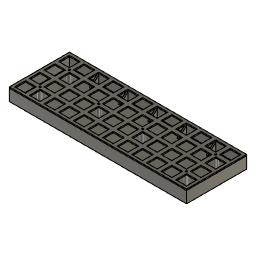
keyboard48 (Autodesk Fusion 360 design; units mm, degrees)
Autodesk Fusion 360 part; units mm, degrees
sketch "Sketch1" plane through (0, 0, 0) normal (0, 0, 1) x (1, 0, 0)
  line L0 (226.5, -3.5) -> (226.5, 74.5)
  line L1 (226.5, 74.5) -> (-3.5, 74.5)
  line L2 (114, 0.05) -> (127.9, 0.05) construction
  line L3 (127.9, 13.95) -> (114, 13.95) construction
  line L4 (223, 64) -> (226.5, 64) construction
  line L5 (206.5, 74.5) -> (206.5, 34.5) construction
  line L6 (199.5, 57.05) -> (213.5, 57.05) construction
  line L7 (213.5, 57.05) -> (213.5, 58.03) construction
  line L8 (213.5, 58.03) -> (215.075, 58.03) construction
  line L9 (215.075, 58.03) -> (215.075, 57.23) construction
  line L10 (215.075, 57.23) -> (216.9, 57.23) construction
  line L11 (216.9, 57.23) -> (216.9, 56.03) construction
  line L12 (216.9, 56.03) -> (219.9, 56.03) construction
  line L13 (219.9, 56.03) -> (219.9, 57.23) construction
  line L14 (219.9, 57.23) -> (221.725, 57.23) construction
  line L15 (221.725, 57.23) -> (221.725, 63.5) construction
  line L16 (221.725, 63.5) -> (222.6, 63.5) construction
  line L17 (222.6, 63.5) -> (222.6, 66.3) construction
  line L18 (222.6, 66.3) -> (221.725, 66.3) construction
  line L19 (221.725, 66.3) -> (221.725, 69.53) construction
  line L20 (221.725, 69.53) -> (215.075, 69.53) construction
  line L21 (215.075, 69.53) -> (215.075, 68.73) construction
  line L22 (215.075, 68.73) -> (213.5, 68.73) construction
  line L23 (213.5, 68.73) -> (213.5, 70.95) construction
  line L24 (213.5, 70.95) -> (199.5, 70.95) construction
  line L25 (199.5, 70.95) -> (199.5, 68.73) construction
  line L26 (199.5, 68.73) -> (197.925, 68.73) construction
  line L27 (197.925, 68.73) -> (197.925, 69.53) construction
  line L28 (197.925, 69.53) -> (191.275, 69.53) construction
  line L29 (191.275, 69.53) -> (191.275, 66.3) construction
  line L30 (190.4, 66.3) -> (190.4, 63.5) construction
  line L31 (190.4, 63.5) -> (191.275, 63.5) construction
  line L32 (191.275, 63.5) -> (191.275, 57.23) construction
  line L33 (191.275, 57.23) -> (193.1, 57.23) construction
  line L34 (193.1, 57.23) -> (193.1, 56.03) construction
  line L35 (193.1, 56.03) -> (196.1, 56.03) construction
  line L36 (196.1, 56.03) -> (196.1, 57.23) construction
  line L37 (196.1, 57.23) -> (197.925, 57.23) construction
  line L38 (197.925, 57.23) -> (197.925, 58.03) construction
  line L39 (197.925, 58.03) -> (199.5, 58.03) construction
  line L40 (199.5, 58.03) -> (199.5, 57.05) construction
  line L41 (190.4, 66.3) -> (191.275, 66.3) construction
  line L42 (199.5, 49.73) -> (197.925, 49.73) construction
  line L43 (215.075, 38.23) -> (216.9, 38.23) construction
  line L44 (213.5, 39.03) -> (215.075, 39.03) construction
  line L45 (213.5, 38.05) -> (213.5, 39.03) construction
  line L46 (215.075, 49.73) -> (213.5, 49.73) construction
  line L47 (213.5, 51.95) -> (199.5, 51.95) construction
  line L48 (199.5, 38.05) -> (213.5, 38.05) construction
  line L49 (193.1, 37.03) -> (196.1, 37.03) construction
  line L50 (191.275, 38.23) -> (193.1, 38.23) construction
  line L51 (197.925, 39.03) -> (199.5, 39.03) construction
  line L52 (222.6, 44.5) -> (222.6, 47.3) construction
  line L53 (221.725, 44.5) -> (222.6, 44.5) construction
  line L54 (199.5, 39.03) -> (199.5, 38.05) construction
  line L55 (191.275, 44.5) -> (191.275, 38.23) construction
  line L56 (196.1, 37.03) -> (196.1, 38.23) construction
  line L57 (221.725, 50.53) -> (215.075, 50.53) construction
  line L58 (196.1, 38.23) -> (197.925, 38.23) construction
  line L59 (215.075, 39.03) -> (215.075, 38.23) construction
  line L60 (197.925, 38.23) -> (197.925, 39.03) construction
  line L61 (197.925, 50.53) -> (191.275, 50.53) construction
  line L62 (216.9, 38.23) -> (216.9, 37.03) construction
  line L63 (191.275, 50.53) -> (191.275, 47.3) construction
  line L64 (190.4, 47.3) -> (191.275, 47.3) construction
  line L65 (199.5, 51.95) -> (199.5, 49.73) construction
  line L66 (197.925, 49.73) -> (197.925, 50.53) construction
  line L67 (219.9, 38.23) -> (221.725, 38.23) construction
  line L68 (215.075, 50.53) -> (215.075, 49.73) construction
  line L69 (193.1, 38.23) -> (193.1, 37.03) construction
  line L70 (219.9, 37.03) -> (219.9, 38.23) construction
  line L71 (221.725, 38.23) -> (221.725, 44.5) construction
  line L72 (190.4, 44.5) -> (191.275, 44.5) construction
  line L73 (190.4, 47.3) -> (190.4, 44.5) construction
  line L74 (222.6, 47.3) -> (221.725, 47.3) construction
  line L75 (213.5, 49.73) -> (213.5, 51.95) construction
  line L76 (216.9, 37.03) -> (219.9, 37.03) construction
  line L77 (221.725, 47.3) -> (221.725, 50.53) construction
  line L78 (114, 13.95) -> (114, 8.45) construction
  line L79 (114, 8.45) -> (94.3177, 8.45) construction
  line L80 (94.3177, 8.45) -> (94.3177, 12.6396) construction
  line L81 (94.3177, 12.6396) -> (87.6629, 12.6396) construction
  line L82 (87.6629, 12.6396) -> (87.6629, 9.244) construction
  line L83 (87.6629, 9.244) -> (86.7993, 9.244) construction
  line L84 (86.7993, 9.244) -> (86.7993, 6.45) construction
  line L85 (86.7993, 6.45) -> (87.6629, 6.45) construction
  line L86 (87.6629, 6.45) -> (87.6629, 0.346) construction
  line L87 (87.6629, 0.346) -> (89.4663, 0.346) construction
  line L88 (89.4663, 0.346) -> (89.4663, -0.8224) construction
  line L89 (89.4663, -0.8224) -> (92.5143, -0.8224) construction
  line L90 (92.5143, -0.8224) -> (92.5143, 0.346) construction
  line L91 (92.5143, 0.346) -> (94.3177, 0.346) construction
  line L92 (94.3177, 0.346) -> (94.3177, 5.45) construction
  line L93 (94.3177, 5.45) -> (114, 5.45) construction
  line L94 (114, 5.45) -> (114, 0.05) construction
  line L95 (127.9, 13.95) -> (127.9, 8.45) construction
  line L96 (127.9, 8.45) -> (147.5823, 8.45) construction
  line L97 (147.5823, 8.45) -> (147.5823, 12.6396) construction
  line L98 (147.5823, 12.6396) -> (154.2371, 12.6396) construction
  line L99 (154.2371, 12.6396) -> (154.2371, 9.244) construction
  line L100 (154.2371, 9.244) -> (155.1007, 9.244) construction
  line L101 (155.1007, 9.244) -> (155.1007, 6.45) construction
  line L102 (155.1007, 6.45) -> (154.2371, 6.45) construction
  line L103 (154.2371, 6.45) -> (154.2371, 0.346) construction
  line L104 (154.2371, 0.346) -> (152.4337, 0.346) construction
  line L105 (152.4337, 0.346) -> (152.4337, -0.8224) construction
  line L106 (152.4337, -0.8224) -> (149.3857, -0.8224) construction
  line L107 (149.3857, -0.8224) -> (149.3857, 0.346) construction
  line L108 (149.3857, 0.346) -> (147.5823, 0.346) construction
  line L109 (147.5823, 0.346) -> (147.5823, 5.45) construction
  line L110 (147.5823, 5.45) -> (127.9, 5.45) construction
  line L111 (127.9, 5.45) -> (127.9, 0.05) construction
  line L112 (71, 6.95) -> (171, 6.95) construction
  line L113 (120.95, 19) -> (120.95, -2.5) construction
  line L114 (90.9903, 16.3311) -> (90.9903, -1.1154) construction
  line L115 (150.9097, 15.5) -> (150.9097, -1.5) construction
  line L116 (86.7993, 9.244) -> (90.9903, 9.244) construction
  line L117 (155.1007, 9.244) -> (150.9097, 9.244) construction
  line L118 (-3.5, 74.5) -> (-3.5, -3.5)
  line L119 (-3.5, -3.5) -> (226.5, -3.5)
  line L120 (0, 0) -> (13.9, 0)
  line L121 (13.9, 0) -> (13.9, 13.9)
  line L122 (13.9, 13.9) -> (0, 13.9)
  line L123 (0, 13.9) -> (0, 0)
  line L124 (-1.5, 72.5) -> (224.5, 72.5)
  line L125 (224.5, 72.5) -> (224.5, -1.5)
  line L126 (224.5, -1.5) -> (-1.5, -1.5)
  line L127 (-1.5, -1.5) -> (-1.5, 72.5)
  dimension "d15" = 14
  dimension "d16" = 6.95
  dimension "d17" = 17.15
  dimension "d18" = 20.8
  dimension "d19" = 26.8
  dimension "d20" = 6.95
  dimension "d21" = 30.45
  dimension "d22" = 32.2
  dimension "d23" = 0.5
  dimension "d24" = 2.3
  dimension "d25" = 5.97
  dimension "d26" = 6.77
  dimension "d27" = 7.97
  dimension "d28" = 4.73
  dimension "d29" = 5.53
  dimension "d32" = 0
  dimension "d33" = -19
  dimension "d34" = 7
  dimension "d35" = 13.9
  dimension "d36" = 13.9
  dimension "d37" = 6.6548
  dimension "d38" = 3.048
  dimension "d39" = 2.794
  dimension "d40" = 4.191
  dimension "d41" = 12.2936
  dimension "d42" = 13.462
  dimension "d43" = 6.604
  dimension "d44" = 0.5
  dimension "d45" = 59.9194
  dimension "d46" = 3
  dimension "d86" = 6.95
  dimension "d87" = 120.95
  dimension "d88" = 20
  dimension "d89" = 10.5
  dimension "d90" = 3.5
  dimension "d91" = 3.5
  dimension "d92" = 230
  dimension "d93" = 78
  dimension "d142" = 13.9
  dimension "d143" = 13.9
  dimension "d155" = 2
  dimension "d156" = 2
  dimension "d157" = 2
  dimension "d158" = 2
  constraint coincident L0 L4.end
  constraint perpendicular L0 L4
  constraint coincident L1 L5.start
  constraint perpendicular L1 L5
  constraint perpendicular L5 L6
  constraint symmetric L5 L6.start L6.end
  constraint perpendicular L6 L7
  constraint perpendicular L7 L8
  constraint perpendicular L8 L9
  constraint perpendicular L9 L10
  constraint perpendicular L10 L11
  constraint perpendicular L11 L12
  constraint perpendicular L10 L13
  constraint perpendicular L13 L14
  constraint perpendicular L14 L15
  constraint perpendicular L13 L16
  constraint perpendicular L4 L17
  constraint perpendicular L17 L18
  constraint perpendicular L4 L19
  constraint perpendicular L19 L20
  constraint vertical L8.end L20.end
  constraint perpendicular L20 L21
  constraint perpendicular L7 L22
  constraint perpendicular L4 L23
  constraint perpendicular L23 L24
  constraint perpendicular L22 L25
  constraint perpendicular L5 L26
  constraint perpendicular L22 L27
  constraint perpendicular L5 L28
  constraint perpendicular L22 L29
  constraint perpendicular L4 L30
  constraint perpendicular L29 L31
  constraint perpendicular L4 L32
  constraint perpendicular L32 L33
  constraint perpendicular L4 L34
  constraint perpendicular L34 L35
  constraint perpendicular L4 L36
  constraint perpendicular L34 L37
  constraint perpendicular L4 L38
  constraint perpendicular L34 L39
  constraint perpendicular L6 L40
  constraint symmetric L5 L9 L38
  constraint symmetric L5 L11 L36
  constraint symmetric L5 L13 L34
  constraint perpendicular L29 L41
  constraint equal L6 L24
  constraint collinear L7 L23
  constraint collinear L27 L38
  constraint collinear L29 L32
  constraint collinear L10 L14
  constraint collinear L8 L39
  constraint collinear L10 L37
  constraint collinear L12 L35
  constraint collinear L14 L33
  constraint collinear L16 L31
  constraint collinear L18 L41
  constraint collinear L20 L28
  constraint collinear L22 L26
  constraint perpendicular L3 L78
  constraint perpendicular L78 L79
  constraint perpendicular L3 L80
  constraint perpendicular L80 L81
  constraint perpendicular L81 L82
  constraint perpendicular L82 L83
  constraint perpendicular L83 L84
  constraint perpendicular L82 L85
  constraint perpendicular L85 L86
  constraint perpendicular L82 L87
  constraint perpendicular L85 L88
  constraint perpendicular L82 L89
  constraint perpendicular L89 L90
  constraint perpendicular L80 L91
  constraint perpendicular L91 L92
  constraint perpendicular L78 L93
  constraint perpendicular L2 L94
  constraint perpendicular L79 L95
  constraint perpendicular L78 L96
  constraint perpendicular L96 L97
  constraint perpendicular L97 L98
  constraint perpendicular L98 L99
  constraint perpendicular L97 L100
  constraint perpendicular L98 L101
  constraint perpendicular L101 L102
  constraint perpendicular L102 L103
  constraint perpendicular L103 L104
  constraint perpendicular L102 L105
  constraint perpendicular L105 L106
  constraint perpendicular L106 L107
  constraint perpendicular L107 L108
  constraint perpendicular L96 L109
  constraint perpendicular L109 L110
  constraint perpendicular L2 L111
  constraint collinear L95 L111
  constraint collinear L78 L94
  constraint collinear L79 L96
  constraint collinear L93 L110
  constraint collinear L82 L86
  constraint collinear L80 L92
  constraint vertical L114
  constraint symmetric L88 L90 L114
  constraint equal L84 L101
  constraint equal L81 L98
  constraint equal L89 L106
  constraint collinear L97 L109
  constraint collinear L99 L103
  constraint coincident L114 L116.end
  constraint perpendicular L114 L116
  constraint coincident L115 L117.end
  constraint perpendicular L115 L117
  constraint equal L116 L117
  constraint collinear L104 L108
  constraint collinear L81 L98
  constraint collinear L91 L108
  constraint collinear L89 L106
  constraint collinear L87 L91
  constraint collinear L85 L102
  constraint symmetric L78 L95 L113
  constraint symmetric L79 L93 L112
  constraint perpendicular L112 L118
  constraint horizontal L1
  constraint symmetric L5 L63 L77
  constraint symmetric L5 L52 L73
  constraint symmetric L5 L55 L71
  constraint horizontal L120
  constraint vertical L121
  constraint horizontal L122
  constraint vertical L123
  constraint coincident L120.start L123.end
  constraint horizontal L124
  constraint vertical L125
  constraint horizontal L126
  constraint vertical L127
  measures "d15" distance of L6.start L6.end
  measures "d16" distance of L4 L6
  measures "d17" distance of L9 L38
  measures "d18" distance of L11 L36
  measures "d19" distance of L13 L34
  measures "d20" distance of L4 L24
  measures "d21" distance of L19 L29
  measures "d22" distance of L17 L30
  measures "d23" distance of L4 L16
  measures "d24" distance of L4 L18
  measures "d25" distance of L4 L8
  measures "d26" distance of L4 L14
  measures "d27" distance of L4 L12
  measures "d28" distance of L4 L22
  measures "d29" distance of L4 L20
  measures "d34" distance of L3 L112
  measures "d35" distance of L2 L3
  measures "d36" distance of L94 L111
  measures "d37" distance of L80.end L81.end
  measures "d38" distance of L88.end L89.end
  measures "d39" distance of L83.end L84.end
  measures "d40" distance of L84 L114
  measures "d41" distance of L98 L104
  measures "d42" distance of L98 L106
  measures "d43" distance of L104 L112
  measures "d44" distance of L102 L112
  measures "d45" distance of L114 L115
  measures "d46" distance of L79 L93
  measures "d86" distance of L120.start L112
  measures "d87" distance of L120.start L113
  measures "d88" distance of L0 L5
  measures "d89" distance of L1 L4
  measures "d90" distance of L120.start L119
  measures "d91" distance of L120.start L118
  measures "d92" distance of L0.end L1.end
  measures "d93" distance of L1 L119
  measures "d142" distance of L121.end L122.end
  measures "d143" distance of L120.end L121.end
  measures "d155" distance of L0 L125
  measures "d156" distance of L119 L126
  measures "d157" distance of L1 L124
  measures "d158" distance of L118 L127
extrude "Extrude1" add sketch "Sketch1" along normal blind 1.524 contours L0 L1 L118 L119 | L124 L125 L126 L127 makes body 1
pattern_linear "R-Pattern1" count 12 spacing 19 along (1, 0, 0) count 4 spacing 19 along (0, 1, 0) of 4 faces at (4.6333, 0, 1.016) (13.9, 4.6333, 1.016) (0, 9.2667, 1.016) (9.2667, 13.9, 1.016) on bodies 1
sketch "Sketch4" plane through (0, 0, 0) normal (0, 0, -1) x (1, 0, 0)
  line L0 (226.5, 3.5) -> (-3.5, 3.5)
  line L1 (-3.5, 3.5) -> (-3.5, -74.5)
  line L2 (-3.5, -74.5) -> (226.5, -74.5)
  line L3 (226.5, -74.5) -> (226.5, 3.5)
  line L4 (-1.5, 1.5) -> (228.5, 1.5)
  line L5 (228.5, 1.5) -> (228.5, -76.5)
  line L6 (228.5, -76.5) -> (-1.5, -76.5)
  line L7 (-1.5, -76.5) -> (-1.5, 1.5)
  line L8 (209, -57) -> (222.9, -57)
  line L9 (222.9, -57) -> (222.9, -70.9)
  line L10 (222.9, -70.9) -> (209, -70.9)
  line L11 (209, -70.9) -> (209, -57)
  line L12 (190, -57) -> (203.9, -57)
  line L13 (203.9, -57) -> (203.9, -70.9)
  line L14 (203.9, -70.9) -> (190, -70.9)
  line L15 (190, -70.9) -> (190, -57)
  line L16 (171, -57) -> (184.9, -57)
  line L17 (184.9, -57) -> (184.9, -70.9)
  line L18 (184.9, -70.9) -> (171, -70.9)
  line L19 (171, -70.9) -> (171, -57)
  line L20 (152, -57) -> (165.9, -57)
  line L21 (165.9, -57) -> (165.9, -70.9)
  line L22 (165.9, -70.9) -> (152, -70.9)
  line L23 (152, -70.9) -> (152, -57)
  line L24 (133, -57) -> (146.9, -57)
  line L25 (146.9, -57) -> (146.9, -70.9)
  line L26 (146.9, -70.9) -> (133, -70.9)
  line L27 (133, -70.9) -> (133, -57)
  line L28 (114, -57) -> (127.9, -57)
  line L29 (127.9, -57) -> (127.9, -70.9)
  line L30 (127.9, -70.9) -> (114, -70.9)
  line L31 (114, -70.9) -> (114, -57)
  line L32 (95, -57) -> (108.9, -57)
  line L33 (108.9, -57) -> (108.9, -70.9)
  line L34 (108.9, -70.9) -> (95, -70.9)
  line L35 (95, -70.9) -> (95, -57)
  line L36 (76, -57) -> (89.9, -57)
  line L37 (89.9, -57) -> (89.9, -70.9)
  line L38 (89.9, -70.9) -> (76, -70.9)
  line L39 (76, -70.9) -> (76, -57)
  line L40 (57, -57) -> (70.9, -57)
  line L41 (70.9, -57) -> (70.9, -70.9)
  line L42 (70.9, -70.9) -> (57, -70.9)
  line L43 (57, -70.9) -> (57, -57)
  line L44 (38, -57) -> (51.9, -57)
  line L45 (51.9, -57) -> (51.9, -70.9)
  line L46 (51.9, -70.9) -> (38, -70.9)
  line L47 (38, -70.9) -> (38, -57)
  line L48 (19, -57) -> (32.9, -57)
  line L49 (32.9, -57) -> (32.9, -70.9)
  line L50 (32.9, -70.9) -> (19, -70.9)
  line L51 (19, -70.9) -> (19, -57)
  line L52 (0, -57) -> (13.9, -57)
  line L53 (13.9, -57) -> (13.9, -70.9)
  line L54 (13.9, -70.9) -> (0, -70.9)
  line L55 (0, -70.9) -> (0, -57)
  line L56 (209, -38) -> (222.9, -38)
  line L57 (222.9, -38) -> (222.9, -51.9)
  line L58 (222.9, -51.9) -> (209, -51.9)
  line L59 (209, -51.9) -> (209, -38)
  line L60 (190, -38) -> (203.9, -38)
  line L61 (203.9, -38) -> (203.9, -51.9)
  line L62 (203.9, -51.9) -> (190, -51.9)
  line L63 (190, -51.9) -> (190, -38)
  line L64 (171, -38) -> (184.9, -38)
  line L65 (184.9, -38) -> (184.9, -51.9)
  line L66 (184.9, -51.9) -> (171, -51.9)
  line L67 (171, -51.9) -> (171, -38)
  line L68 (152, -38) -> (165.9, -38)
  line L69 (165.9, -38) -> (165.9, -51.9)
  line L70 (165.9, -51.9) -> (152, -51.9)
  line L71 (152, -51.9) -> (152, -38)
  line L72 (133, -38) -> (146.9, -38)
  line L73 (146.9, -38) -> (146.9, -51.9)
  line L74 (146.9, -51.9) -> (133, -51.9)
  line L75 (133, -51.9) -> (133, -38)
  line L76 (114, -38) -> (127.9, -38)
  line L77 (127.9, -38) -> (127.9, -51.9)
  line L78 (127.9, -51.9) -> (114, -51.9)
  line L79 (114, -51.9) -> (114, -38)
  line L80 (95, -38) -> (108.9, -38)
  line L81 (108.9, -38) -> (108.9, -51.9)
  line L82 (108.9, -51.9) -> (95, -51.9)
  line L83 (95, -51.9) -> (95, -38)
  line L84 (76, -38) -> (89.9, -38)
  line L85 (89.9, -38) -> (89.9, -51.9)
  line L86 (89.9, -51.9) -> (76, -51.9)
  line L87 (76, -51.9) -> (76, -38)
  line L88 (57, -38) -> (70.9, -38)
  line L89 (70.9, -38) -> (70.9, -51.9)
  line L90 (70.9, -51.9) -> (57, -51.9)
  line L91 (57, -51.9) -> (57, -38)
  line L92 (38, -38) -> (51.9, -38)
  line L93 (51.9, -38) -> (51.9, -51.9)
  line L94 (51.9, -51.9) -> (38, -51.9)
  line L95 (38, -51.9) -> (38, -38)
  line L96 (19, -38) -> (32.9, -38)
  line L97 (32.9, -38) -> (32.9, -51.9)
  line L98 (32.9, -51.9) -> (19, -51.9)
  line L99 (19, -51.9) -> (19, -38)
  line L100 (0, -38) -> (13.9, -38)
  line L101 (13.9, -38) -> (13.9, -51.9)
  line L102 (13.9, -51.9) -> (0, -51.9)
  line L103 (0, -51.9) -> (0, -38)
  line L104 (209, -19) -> (222.9, -19)
  line L105 (222.9, -19) -> (222.9, -32.9)
  line L106 (222.9, -32.9) -> (209, -32.9)
  line L107 (209, -32.9) -> (209, -19)
  line L108 (190, -19) -> (203.9, -19)
  line L109 (203.9, -19) -> (203.9, -32.9)
  line L110 (203.9, -32.9) -> (190, -32.9)
  line L111 (190, -32.9) -> (190, -19)
  line L112 (171, -19) -> (184.9, -19)
  line L113 (184.9, -19) -> (184.9, -32.9)
  line L114 (184.9, -32.9) -> (171, -32.9)
  line L115 (171, -32.9) -> (171, -19)
  line L116 (152, -19) -> (165.9, -19)
  line L117 (165.9, -19) -> (165.9, -32.9)
  line L118 (165.9, -32.9) -> (152, -32.9)
  line L119 (152, -32.9) -> (152, -19)
  line L120 (133, -19) -> (146.9, -19)
  line L121 (146.9, -19) -> (146.9, -32.9)
  line L122 (146.9, -32.9) -> (133, -32.9)
  line L123 (133, -32.9) -> (133, -19)
  line L124 (114, -19) -> (127.9, -19)
  line L125 (127.9, -19) -> (127.9, -32.9)
  line L126 (127.9, -32.9) -> (114, -32.9)
  line L127 (114, -32.9) -> (114, -19)
  line L128 (95, -19) -> (108.9, -19)
  line L129 (108.9, -19) -> (108.9, -32.9)
  line L130 (108.9, -32.9) -> (95, -32.9)
  line L131 (95, -32.9) -> (95, -19)
  line L132 (76, -19) -> (89.9, -19)
  line L133 (89.9, -19) -> (89.9, -32.9)
  line L134 (89.9, -32.9) -> (76, -32.9)
  line L135 (76, -32.9) -> (76, -19)
  line L136 (57, -19) -> (70.9, -19)
  line L137 (70.9, -19) -> (70.9, -32.9)
  line L138 (70.9, -32.9) -> (57, -32.9)
  line L139 (57, -32.9) -> (57, -19)
  line L140 (38, -19) -> (51.9, -19)
  line L141 (51.9, -19) -> (51.9, -32.9)
  line L142 (51.9, -32.9) -> (38, -32.9)
  line L143 (38, -32.9) -> (38, -19)
  line L144 (19, -19) -> (32.9, -19)
  line L145 (32.9, -19) -> (32.9, -32.9)
  line L146 (32.9, -32.9) -> (19, -32.9)
  line L147 (19, -32.9) -> (19, -19)
  line L148 (0, -19) -> (13.9, -19)
  line L149 (13.9, -19) -> (13.9, -32.9)
  line L150 (13.9, -32.9) -> (0, -32.9)
  line L151 (0, -32.9) -> (0, -19)
  line L152 (209, 0) -> (222.9, 0)
  line L153 (222.9, 0) -> (222.9, -13.9)
  line L154 (222.9, -13.9) -> (209, -13.9)
  line L155 (209, -13.9) -> (209, 0)
  line L156 (190, 0) -> (203.9, 0)
  line L157 (203.9, 0) -> (203.9, -13.9)
  line L158 (203.9, -13.9) -> (190, -13.9)
  line L159 (190, -13.9) -> (190, 0)
  line L160 (171, 0) -> (184.9, 0)
  line L161 (184.9, 0) -> (184.9, -13.9)
  line L162 (184.9, -13.9) -> (171, -13.9)
  line L163 (171, -13.9) -> (171, 0)
  line L164 (152, 0) -> (165.9, 0)
  line L165 (165.9, 0) -> (165.9, -13.9)
  line L166 (165.9, -13.9) -> (152, -13.9)
  line L167 (152, -13.9) -> (152, 0)
  line L168 (133, 0) -> (146.9, 0)
  line L169 (146.9, 0) -> (146.9, -13.9)
  line L170 (146.9, -13.9) -> (133, -13.9)
  line L171 (133, -13.9) -> (133, 0)
  line L172 (114, 0) -> (127.9, 0)
  line L173 (127.9, 0) -> (127.9, -13.9)
  line L174 (127.9, -13.9) -> (114, -13.9)
  line L175 (114, -13.9) -> (114, 0)
  line L176 (95, 0) -> (108.9, 0)
  line L177 (108.9, 0) -> (108.9, -13.9)
  line L178 (108.9, -13.9) -> (95, -13.9)
  line L179 (95, -13.9) -> (95, 0)
  line L180 (76, 0) -> (89.9, 0)
  line L181 (89.9, 0) -> (89.9, -13.9)
  line L182 (89.9, -13.9) -> (76, -13.9)
  line L183 (76, -13.9) -> (76, 0)
  line L184 (57, 0) -> (70.9, 0)
  line L185 (70.9, 0) -> (70.9, -13.9)
  line L186 (70.9, -13.9) -> (57, -13.9)
  line L187 (57, -13.9) -> (57, 0)
  line L188 (38, 0) -> (51.9, 0)
  line L189 (51.9, 0) -> (51.9, -13.9)
  line L190 (51.9, -13.9) -> (38, -13.9)
  line L191 (38, -13.9) -> (38, 0)
  line L192 (19, 0) -> (32.9, 0)
  line L193 (32.9, 0) -> (32.9, -13.9)
  line L194 (32.9, -13.9) -> (19, -13.9)
  line L195 (19, -13.9) -> (19, 0)
  line L196 (0, -13.9) -> (0, 0)
  line L197 (0, 0) -> (13.9, 0)
  line L198 (13.9, 0) -> (13.9, -13.9)
  line L199 (13.9, -13.9) -> (0, -13.9)
  dimension "d82" = 2
  dimension "d83" = 2
  dimension "d84" = 2
  dimension "d85" = 2
  constraint horizontal L4
  constraint vertical L5
  constraint horizontal L6
  constraint vertical L7
  measures "d82" distance of L3 L5
  measures "d83" distance of L2 L6
  measures "d84" distance of L0 L4
  measures "d85" distance of L1 L7
sketch "Sketch1 (2)" plane through (0, 0, 0) normal (0, 0, -1) x (1, 0, 0) in component "pool"
  line L0 (226.5, 3.5) -> (-3.5, 3.5)
  line L1 (-3.5, 3.5) -> (-3.5, -74.5)
  line L2 (-3.5, -74.5) -> (226.5, -74.5)
  line L3 (226.5, -74.5) -> (226.5, 3.5)
  line L4 (-1.5, 1.5) -> (224.5, 1.5)
  line L5 (224.5, 1.5) -> (224.5, -72.5)
  line L6 (224.5, -72.5) -> (-1.5, -72.5)
  line L7 (-1.5, -72.5) -> (-1.5, 1.5)
  line L8 (209, -57) -> (222.9, -57)
  line L9 (222.9, -57) -> (222.9, -70.9)
  line L10 (222.9, -70.9) -> (209, -70.9)
  line L11 (209, -70.9) -> (209, -57)
  line L12 (190, -57) -> (203.9, -57)
  line L13 (203.9, -57) -> (203.9, -70.9)
  line L14 (203.9, -70.9) -> (190, -70.9)
  line L15 (190, -70.9) -> (190, -57)
  line L16 (171, -57) -> (184.9, -57)
  line L17 (184.9, -57) -> (184.9, -70.9)
  line L18 (184.9, -70.9) -> (171, -70.9)
  line L19 (171, -70.9) -> (171, -57)
  line L20 (152, -57) -> (165.9, -57)
  line L21 (165.9, -57) -> (165.9, -70.9)
  line L22 (165.9, -70.9) -> (152, -70.9)
  line L23 (152, -70.9) -> (152, -57)
  line L24 (133, -57) -> (146.9, -57)
  line L25 (146.9, -57) -> (146.9, -70.9)
  line L26 (146.9, -70.9) -> (133, -70.9)
  line L27 (133, -70.9) -> (133, -57)
  line L28 (114, -57) -> (127.9, -57)
  line L29 (127.9, -57) -> (127.9, -70.9)
  line L30 (127.9, -70.9) -> (114, -70.9)
  line L31 (114, -70.9) -> (114, -57)
  line L32 (95, -57) -> (108.9, -57)
  line L33 (108.9, -57) -> (108.9, -70.9)
  line L34 (108.9, -70.9) -> (95, -70.9)
  line L35 (95, -70.9) -> (95, -57)
  line L36 (76, -57) -> (89.9, -57)
  line L37 (89.9, -57) -> (89.9, -70.9)
  line L38 (89.9, -70.9) -> (76, -70.9)
  line L39 (76, -70.9) -> (76, -57)
  line L40 (57, -57) -> (70.9, -57)
  line L41 (70.9, -57) -> (70.9, -70.9)
  line L42 (70.9, -70.9) -> (57, -70.9)
  line L43 (57, -70.9) -> (57, -57)
  line L44 (38, -57) -> (51.9, -57)
  line L45 (51.9, -57) -> (51.9, -70.9)
  line L46 (51.9, -70.9) -> (38, -70.9)
  line L47 (38, -70.9) -> (38, -57)
  line L48 (19, -57) -> (32.9, -57)
  line L49 (32.9, -57) -> (32.9, -70.9)
  line L50 (32.9, -70.9) -> (19, -70.9)
  line L51 (19, -70.9) -> (19, -57)
  line L52 (0, -57) -> (13.9, -57)
  line L53 (13.9, -57) -> (13.9, -70.9)
  line L54 (13.9, -70.9) -> (0, -70.9)
  line L55 (0, -70.9) -> (0, -57)
  line L56 (209, -38) -> (222.9, -38)
  line L57 (222.9, -38) -> (222.9, -51.9)
  line L58 (222.9, -51.9) -> (209, -51.9)
  line L59 (209, -51.9) -> (209, -38)
  line L60 (190, -38) -> (203.9, -38)
  line L61 (203.9, -38) -> (203.9, -51.9)
  line L62 (203.9, -51.9) -> (190, -51.9)
  line L63 (190, -51.9) -> (190, -38)
  line L64 (171, -38) -> (184.9, -38)
  line L65 (184.9, -38) -> (184.9, -51.9)
  line L66 (184.9, -51.9) -> (171, -51.9)
  line L67 (171, -51.9) -> (171, -38)
  line L68 (152, -38) -> (165.9, -38)
  line L69 (165.9, -38) -> (165.9, -51.9)
  line L70 (165.9, -51.9) -> (152, -51.9)
  line L71 (152, -51.9) -> (152, -38)
  line L72 (133, -38) -> (146.9, -38)
  line L73 (146.9, -38) -> (146.9, -51.9)
  line L74 (146.9, -51.9) -> (133, -51.9)
  line L75 (133, -51.9) -> (133, -38)
  line L76 (114, -38) -> (127.9, -38)
  line L77 (127.9, -38) -> (127.9, -51.9)
  line L78 (127.9, -51.9) -> (114, -51.9)
  line L79 (114, -51.9) -> (114, -38)
  line L80 (95, -38) -> (108.9, -38)
  line L81 (108.9, -38) -> (108.9, -51.9)
  line L82 (108.9, -51.9) -> (95, -51.9)
  line L83 (95, -51.9) -> (95, -38)
  line L84 (76, -38) -> (89.9, -38)
  line L85 (89.9, -38) -> (89.9, -51.9)
  line L86 (89.9, -51.9) -> (76, -51.9)
  line L87 (76, -51.9) -> (76, -38)
  line L88 (57, -38) -> (70.9, -38)
  line L89 (70.9, -38) -> (70.9, -51.9)
  line L90 (70.9, -51.9) -> (57, -51.9)
  line L91 (57, -51.9) -> (57, -38)
  line L92 (38, -38) -> (51.9, -38)
  line L93 (51.9, -38) -> (51.9, -51.9)
  line L94 (51.9, -51.9) -> (38, -51.9)
  line L95 (38, -51.9) -> (38, -38)
  line L96 (19, -38) -> (32.9, -38)
  line L97 (32.9, -38) -> (32.9, -51.9)
  line L98 (32.9, -51.9) -> (19, -51.9)
  line L99 (19, -51.9) -> (19, -38)
  line L100 (0, -38) -> (13.9, -38)
  line L101 (13.9, -38) -> (13.9, -51.9)
  line L102 (13.9, -51.9) -> (0, -51.9)
  line L103 (0, -51.9) -> (0, -38)
  line L104 (209, -19) -> (222.9, -19)
  line L105 (222.9, -19) -> (222.9, -32.9)
  line L106 (222.9, -32.9) -> (209, -32.9)
  line L107 (209, -32.9) -> (209, -19)
  line L108 (190, -19) -> (203.9, -19)
  line L109 (203.9, -19) -> (203.9, -32.9)
  line L110 (203.9, -32.9) -> (190, -32.9)
  line L111 (190, -32.9) -> (190, -19)
  line L112 (171, -19) -> (184.9, -19)
  line L113 (184.9, -19) -> (184.9, -32.9)
  line L114 (184.9, -32.9) -> (171, -32.9)
  line L115 (171, -32.9) -> (171, -19)
  line L116 (152, -19) -> (165.9, -19)
  line L117 (165.9, -19) -> (165.9, -32.9)
  line L118 (165.9, -32.9) -> (152, -32.9)
  line L119 (152, -32.9) -> (152, -19)
  line L120 (133, -19) -> (146.9, -19)
  line L121 (146.9, -19) -> (146.9, -32.9)
  line L122 (146.9, -32.9) -> (133, -32.9)
  line L123 (133, -32.9) -> (133, -19)
  line L124 (114, -19) -> (127.9, -19)
  line L125 (127.9, -19) -> (127.9, -32.9)
  line L126 (127.9, -32.9) -> (114, -32.9)
  line L127 (114, -32.9) -> (114, -19)
  line L128 (95, -19) -> (108.9, -19)
  line L129 (108.9, -19) -> (108.9, -32.9)
  line L130 (108.9, -32.9) -> (95, -32.9)
  line L131 (95, -32.9) -> (95, -19)
  line L132 (76, -19) -> (89.9, -19)
  line L133 (89.9, -19) -> (89.9, -32.9)
  line L134 (89.9, -32.9) -> (76, -32.9)
  line L135 (76, -32.9) -> (76, -19)
  line L136 (57, -19) -> (70.9, -19)
  line L137 (70.9, -19) -> (70.9, -32.9)
  line L138 (70.9, -32.9) -> (57, -32.9)
  line L139 (57, -32.9) -> (57, -19)
  line L140 (38, -19) -> (51.9, -19)
  line L141 (51.9, -19) -> (51.9, -32.9)
  line L142 (51.9, -32.9) -> (38, -32.9)
  line L143 (38, -32.9) -> (38, -19)
  line L144 (19, -19) -> (32.9, -19)
  line L145 (32.9, -19) -> (32.9, -32.9)
  line L146 (32.9, -32.9) -> (19, -32.9)
  line L147 (19, -32.9) -> (19, -19)
  line L148 (0, -19) -> (13.9, -19)
  line L149 (13.9, -19) -> (13.9, -32.9)
  line L150 (13.9, -32.9) -> (0, -32.9)
  line L151 (0, -32.9) -> (0, -19)
  line L152 (209, 0) -> (222.9, 0)
  line L153 (222.9, 0) -> (222.9, -13.9)
  line L154 (222.9, -13.9) -> (209, -13.9)
  line L155 (209, -13.9) -> (209, 0)
  line L156 (190, 0) -> (203.9, 0)
  line L157 (203.9, 0) -> (203.9, -13.9)
  line L158 (203.9, -13.9) -> (190, -13.9)
  line L159 (190, -13.9) -> (190, 0)
  line L160 (171, 0) -> (184.9, 0)
  line L161 (184.9, 0) -> (184.9, -13.9)
  line L162 (184.9, -13.9) -> (171, -13.9)
  line L163 (171, -13.9) -> (171, 0)
  line L164 (152, 0) -> (165.9, 0)
  line L165 (165.9, 0) -> (165.9, -13.9)
  line L166 (165.9, -13.9) -> (152, -13.9)
  line L167 (152, -13.9) -> (152, 0)
  line L168 (133, 0) -> (146.9, 0)
  line L169 (146.9, 0) -> (146.9, -13.9)
  line L170 (146.9, -13.9) -> (133, -13.9)
  line L171 (133, -13.9) -> (133, 0)
  line L172 (114, 0) -> (127.9, 0)
  line L173 (127.9, 0) -> (127.9, -13.9)
  line L174 (127.9, -13.9) -> (114, -13.9)
  line L175 (114, -13.9) -> (114, 0)
  line L176 (95, 0) -> (108.9, 0)
  line L177 (108.9, 0) -> (108.9, -13.9)
  line L178 (108.9, -13.9) -> (95, -13.9)
  line L179 (95, -13.9) -> (95, 0)
  line L180 (76, 0) -> (89.9, 0)
  line L181 (89.9, 0) -> (89.9, -13.9)
  line L182 (89.9, -13.9) -> (76, -13.9)
  line L183 (76, -13.9) -> (76, 0)
  line L184 (57, 0) -> (70.9, 0)
  line L185 (70.9, 0) -> (70.9, -13.9)
  line L186 (70.9, -13.9) -> (57, -13.9)
  line L187 (57, -13.9) -> (57, 0)
  line L188 (38, 0) -> (51.9, 0)
  line L189 (51.9, 0) -> (51.9, -13.9)
  line L190 (51.9, -13.9) -> (38, -13.9)
  line L191 (38, -13.9) -> (38, 0)
  line L192 (19, 0) -> (32.9, 0)
  line L193 (32.9, 0) -> (32.9, -13.9)
  line L194 (32.9, -13.9) -> (19, -13.9)
  line L195 (19, -13.9) -> (19, 0)
  line L196 (0, -13.9) -> (0, 0)
  line L197 (0, 0) -> (13.9, 0)
  line L198 (13.9, 0) -> (13.9, -13.9)
  line L199 (13.9, -13.9) -> (0, -13.9)
  line L200 (-3.5, 3.5) -> (226.5, 3.5)
  line L201 (-3.5, -74.5) -> (-3.5, 3.5)
  line L202 (226.5, -74.5) -> (-3.5, -74.5)
  line L203 (226.5, 3.5) -> (226.5, -74.5)
  dimension "d159" = 2
  dimension "d160" = 2
  dimension "d162" = 2
  dimension "d163" = 2
  constraint horizontal L4
  constraint vertical L5
  constraint horizontal L6
  constraint vertical L7
  measures "d159" distance of L4 L200
  measures "d160" distance of L7 L201
  measures "d162" distance of L6 L202
  measures "d163" distance of L5 L203
extrude "Extrude1'" add sketch "Sketch1 (2)" along normal blind 13 separate body contours L0 L1 L2 L3 L200 L201 L202 L203 makes body 2 in component "pool"
sketch "Sketch2" plane through (0, 0, -13) normal (0, 0, -1) x (1, 0, 0) in component "pool"
  line L0 (224.5, -72.5) -> (-1.5, -72.5)
  line L1 (-1.5, -72.5) -> (-1.5, 1.5)
  line L2 (-1.5, 1.5) -> (224.5, 1.5)
  line L3 (224.5, 1.5) -> (224.5, -72.5)
  line L4 (226.5, -74.5) -> (226.5, 3.5)
  line L5 (226.5, 3.5) -> (-3.5, 3.5)
  line L6 (-3.5, 3.5) -> (-3.5, -74.5)
  line L7 (-3.5, -74.5) -> (226.5, -74.5)
  line L8 (-1.5, 1.5) -> (224.5, 1.5)
  line L9 (224.5, 1.5) -> (224.5, -72.5)
  line L10 (224.5, -72.5) -> (-1.5, -72.5)
  line L11 (-1.5, -72.5) -> (-1.5, 1.5)
  constraint horizontal L8
  constraint vertical L9
  constraint horizontal L10
  constraint vertical L11
  constraint coincident L0.start L3.end
  constraint coincident L1.end L2.start
extrude "Extrude2" add sketch "Sketch2" along normal blind 2 contours L0 L1 L2 L3 L8 L9 L10 L11 | L4 L5 L6 L7 bodies 2 in component "pool"
sketch "Sketch3" plane through (0, 0, -13) normal (0, 0, 1) x (-1, 0, 0) in component "pool"
  line L0 (-13.9, -57) -> (-19, -51.9) construction
  line L1 (-19, -51.9) -> (-19, -57) construction
  line L2 (-13.9, -19) -> (-19, -13.9) construction
  line L3 (-19, -13.9) -> (-19, -19) construction
  line L4 (-70.9, -38) -> (-76, -32.9) construction
  line L5 (-76, -32.9) -> (-76, -38) construction
  line L6 (-127.9, -38) -> (-133, -32.9) construction
  line L7 (-133, -32.9) -> (-133, -38) construction
  line L8 (-203.9, -19) -> (-209, -13.9) construction
  line L9 (-209, -13.9) -> (-209, -19) construction
  line L10 (-203.9, -57) -> (-209, -51.9) construction
  line L11 (-209, -51.9) -> (-209, -57) construction
  circle A0 centre (-206.45, -16.45) radius 2.55
  circle A1 centre (-206.45, -54.45) radius 2.55
  circle A2 centre (-130.45, -35.45) radius 2.55
  circle A3 centre (-73.45, -35.45) radius 2.55
  circle A4 centre (-16.45, -16.45) radius 2.55
  circle A5 centre (-16.45, -54.45) radius 2.55
  line L12 (-224.5, 1.5) -> (-224.5, -72.5)
  line L13 (-224.5, -72.5) -> (1.5, -72.5)
  line L14 (1.5, -72.5) -> (1.5, 1.5)
  line L15 (1.5, 1.5) -> (-224.5, 1.5)
  line L16 (-32.9, -38) -> (-38, -32.9) construction
  line L17 (-38, -32.9) -> (-38, -38) construction
  circle A6 centre (-35.45, -35.45) radius 2.55 construction
  circle A7 centre (-16.45, -16.45) radius 0.5
  circle A8 centre (-16.45, -54.45) radius 0.5
  circle A9 centre (-73.45, -35.45) radius 0.5
  circle A10 centre (-130.45, -35.45) radius 0.5
  circle A11 centre (-206.45, -54.45) radius 0.5
  circle A12 centre (-206.45, -16.45) radius 0.5
  point P0 (-13.9, -57)
  point P1 (-19, -57)
  point P2 (-19, -51.9)
  point P3 (-13.9, -19)
  point P4 (-19, -19)
  point P5 (-76, -38)
  point P6 (-70.9, -38)
  point P7 (-76, -32.9)
  point P8 (-133, -38)
  point P9 (-127.9, -38)
  point P10 (-133, -32.9)
  point P11 (-203.9, -57)
  point P12 (-209, -57)
  point P13 (-209, -13.9)
  point P14 (-203.9, -19)
  point P15 (-209, -19)
  point P16 (-32.9, -38)
  point P17 (-38, -38)
  point P18 (-38, -32.9)
  dimension "d169" = 1
  constraint vertical L1
  constraint parallel L0 L2
  constraint parallel L6 L8
  constraint vertical L9
  constraint parallel L8 L10
  constraint parallel L9 L11
  constraint vertical L7
  constraint coincident P0 L0.start
  constraint coincident P1 L1.end
  constraint coincident L0.end L1.start
  constraint coincident P3 L2.start
  constraint coincident P4 L3.end
  constraint coincident P5 L5.end
  constraint coincident P6 L4.start
  constraint coincident P7 L4.end
  constraint coincident P8 L7.end
  constraint coincident P9 L6.start
  constraint coincident P10 L6.end
  constraint coincident P11 L10.start
  constraint coincident P12 L11.end
  constraint coincident P13 L8.end
  constraint coincident P14 L8.start
  constraint coincident L9.end P15
  constraint midpoint L8 A0.centre
  constraint tangent L9 A0
  constraint midpoint L10 A1.centre
  constraint midpoint L6 A2.centre
  constraint tangent L7 A2
  constraint midpoint L4 A3.centre
  constraint tangent L5 A3
  constraint midpoint L2 A4.centre
  constraint tangent L3 A4
  constraint midpoint L0 A5.centre
  constraint tangent L1 A5
  constraint tangent L11 A1
  constraint vertical L17
  constraint coincident P16 L16.start
  constraint coincident P17 L17.end
  constraint coincident P18 L16.end
  constraint midpoint L16 A6.centre
  constraint tangent L17 A6
  constraint concentric A4 A7
  constraint concentric A5 A8
  constraint concentric A3 A9
  constraint concentric A2 A10
  constraint concentric A1 A11
  constraint concentric A0 A12
  constraint equal A10 A12
  constraint equal A9 A10
  constraint equal A8 A9
  constraint equal A7 A8
  constraint equal A11 A12
  measures "d169" diameter of A11
extrude "Extrude3" add sketch "Sketch3" along normal up to surface (13 mm away) separate body contours A0 | A1 | A2 | A3 | A4 | A5 makes body 3 at (72.6379, 33.0328, -4.3333) makes body 4 at (208.4034, 56.0891, -4.3333) makes body 5 at (13.9127, 54.7039, -4.3333) makes body 6 at (130.5136, 32.9008, -4.3333) makes body 7 at (205.6379, 14.0328, -4.3333) makes body 8 at (13.9127, 16.7039, -4.3333) in component "pool"
sketch "Sketch4 (2)" plane through (0, 0, 1.524) normal (0, 0, 1) x (-1, 0, 0) in component "pool"
  circle A0 centre (-16.45, -54.45) radius 0.5
  circle A1 centre (-16.45, -16.45) radius 0.5
  circle A2 centre (-73.45, -35.45) radius 0.5
  circle A3 centre (-130.45, -35.45) radius 0.5
  circle A4 centre (-206.45, -16.45) radius 0.5
  circle A5 centre (-206.45, -54.45) radius 0.5
  point P0 (-16.45, -54.45)
  point P1 (-73.45, -35.45)
  point P2 (-16.45, -16.45)
  point P3 (-130.45, -35.45)
  point P4 (-206.45, -54.45)
  point P5 (-206.45, -16.45)
  point P6 (-16.45, -54.45)
  point P7 (-16.45, -16.45)
  point P8 (-73.45, -35.45)
  point P9 (-130.45, -35.45)
  point P10 (-206.45, -16.45)
  point P11 (-206.45, -54.45)
  dimension "d168" = 1
  constraint coincident P6 P0
  constraint coincident P7 P2
  constraint coincident P8 P1
  constraint coincident P9 P3
  constraint coincident P10 P5
  constraint coincident P11 P4
  constraint equal A2 A3
  constraint equal A1 A2
  constraint equal A2 A4
  constraint equal A4 A5
  constraint equal A0 A2
  measures "d168" diameter of A0
hole "Hole2" at (16.45, 54.45, 1.524) at (16.45, 16.45, 1.524) at (73.45, 35.45, 1.524) at (130.45, 35.45, 1.524) at (206.45, 16.45, 1.524) at (206.45, 54.45, 1.524) direction (0, 0, -1) diameter 1 depth 15 tip angle 118 countersink diameter 2.4 countersink angle 90 bodies 1
hole "Hole1" at (16.45, 54.45, 1.524) at (16.45, 16.45, 1.524) at (73.45, 35.45, 1.524) at (130.45, 35.45, 1.524) at (206.45, 16.45, 1.524) at (206.45, 54.45, 1.524) direction (0, 0, -1) diameter 1 depth 15 tip angle 118 countersink diameter 2.4 countersink angle 90 bodies 2 in component "pool"
ref_plane "WorkPlane1" through (111.5, 35.5, -7.5) normal (-1, 0, 0) x (0, 1, 0) in component "pool"
sketch "Sketch5" plane through (111.5, 83, 0.762) normal (-1, 0, 0) x (0, 1, 0) in component "pool"
  line L0 (-84.5, 0.762) -> (-84.5, 13.762) construction
  line L1 (-84.5, 13.762) -> (-10.5, 13.762) construction
  line L2 (-10.5, 13.762) -> (-10.5, 0.762) construction
  line L3 (-86.5, 0.762) -> (-86.5, 15.762) construction
  line L4 (-8.5, 15.762) -> (-86.5, 15.762) construction
  line L5 (-8.5, 0.762) -> (-8.5, 15.762) construction
  line L6 (-8.5, 0.762) -> (-86.5, 0.762) construction
  line L7 (-84.5, 13.762) -> (-84.5, 3.7445)
  line L8 (-84.5, 13.762) -> (-74.0034, 13.762)
  line L9 (-74.0034, 13.762) -> (-84.5, 3.7445)
  line L10 (-10.5, 13.762) -> (-10.5, 3.7445)
  line L11 (-10.5, 3.7445) -> (-20.9966, 13.762)
  line L12 (-20.9966, 13.762) -> (-10.5, 13.762)
  line L13 (-84.5, 3.7445) -> (-10.5, 3.7445) construction
  dimension "d170" = 2
  dimension "d171" = 2
  dimension "d172" = 2
  constraint vertical L0
  constraint perpendicular L0 L1
  constraint perpendicular L1 L2
  constraint coincident L0.start L6
  constraint coincident L2.end L6
  constraint coincident L0 L7.end
  constraint coincident L1 L8.end
  constraint coincident L2 L10.end
  constraint coincident L1 L11.end
  constraint perpendicular L2 L13
  constraint equal L9 L11
  measures "d170" distance of L0 L3
  measures "d171" distance of L1 L4
  measures "d172" distance of L2 L5
extrude "Extrude4" add sketch "Sketch5" along normal mid plane 2 bodies 2 in component "pool"
pattern_linear "R-Pattern3" count 5 spacing 38 along (-1, 0, 0) both ways of "Extrude4" in component "pool"
component "pool" placed x (1, 0, 0) y (0, 1, 0) z (0, 0, 1) at (0, 0, 0)
equation "d16 = keyHole / 2"
equation "d20 = keyHole / 2"
equation "d35 = keyHole"
equation "d36 = keyHole"
equation "d37 = ( 0.262 * 25.4 ) * 1 mm"
equation "d38 = ( 0.12 * 25.4 ) * 1 mm"
equation "d39 = ( 0.11 * 25.4 ) * 1 mm"
equation "d40 = ( 0.165 * 25.4 ) * 1 mm"
equation "d41 = ( 0.484 * 25.4 ) * 1 mm"
equation "d42 = ( 0.53 * 25.4 ) * 1 mm"
equation "d43 = ( 0.26 * 25.4 ) * 1 mm"
equation "d47 = ( 0.06 * 25.4 ) * 1 mm"
equation "d82 = shellThick"
equation "d83 = shellThick"
equation "d84 = shellThick"
equation "d85 = shellThick"
equation "d86 = d16"
equation "d87 = keyToKey * 6 + keyHole / 2"
equation "d90 = shellThick / 2 + spacing / 2"
equation "d91 = d90"
equation "d92 = keyboardWidth"
equation "d93 = keyboardHeight"
equation "d98 = COLUMNS"
equation "d99 = ROWS"
equation "d100 = keyToKey"
equation "d101 = -keyToKey"
equation "spacing = 5 mm"
equation "keyHole = 13.9 mm"
equation "keyToKey = 19 mm"
equation "shellThick = 2 mm"
equation "d110 = shellThick"
equation "d111 = d110"
equation "d114 = 15 mm - shellThick"
equation "d116 = shellThick"
equation "d126 = shellThick"
equation "d142 = keyHole"
equation "d143 = keyHole"
equation "ROWS = 4"
equation "keyboardHeight = keyToKey * ROWS + shellThick"
equation "COLUMNS = 12"
equation "keyboardWidth = keyToKey * COLUMNS + shellThick"
equation "d155 = shellThick"
equation "d156 = shellThick"
equation "d157 = shellThick"
equation "d158 = shellThick"
equation "d159 = shellThick"
equation "d160 = shellThick"
equation "d162 = shellThick"
equation "d163 = shellThick"
equation "d170 = shellThick"
equation "d171 = shellThick"
equation "d172 = shellThick"
equation "d175 = -keyToKey * 2"
named bodies: "plate"
